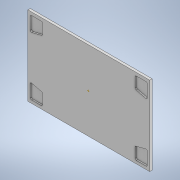
# Autodesk Inventor part: enclosuret
Saved by Autodesk Inventor 2021 (Build 250183000, 183)
## iProperties
Created: 2020-12-16
Part Number: enclosuret
Material: Generic
Document SubType Name: Modeling
Designer: oskar
Density: 1 g/cm^3
Appearance: Default
Author: oskar
Autodesk Inventor part; units mm, degrees
ref_plane "YZ Plane" through (0, 0, 0) normal (1, 0, 0) x (0, 1, 0)
ref_plane "XZ Plane" through (0, 0, 0) normal (0, 1, 0) x (-1, 0, 0)
ref_plane "XY Plane" through (0, 0, 0) normal (0, 0, 1) x (1, 0, 0)
ref_plane "Work Plane1" through (-0.485, 4.902, 12.06) normal (0, 0, 1) x (1, 0, 0)
sketch "Sketch1" plane through (-0.485, 4.902, 12.06) normal (0, 0, 1) x (1, 0, 0)
  line L0 (-52.815, 27.598) -> (47.185, 27.598)
  line L1 (47.185, 27.598) -> (47.185, -37.402)
  line L2 (47.185, -37.402) -> (-52.815, -37.402)
  line L3 (-52.815, -37.402) -> (-52.815, 27.598)
  line L4 (-52.815, 27.598) -> (47.185, -37.402) construction
  line L5 (47.185, 27.598) -> (-52.815, -37.402) construction
  line L6 (46.185, -13.982) -> (46.185, -20.322) projected
  line L7 (0.485, -4.902) -> (-19.0054, -4.902) construction
  point P0 (-2.815, -4.902)
  point P1 (-2.815, -4.902)
  dimension "d0" = 100
  dimension "d1" = 65
  dimension "d2" = 1
  constraints: 14 end point, 3 midpoint, 2 horizontal, 2 parallel, 1 perpendicular, 1 point on line
  measures "d0" distance of L0.start L0.end
  measures "d1" distance of L2.end L0.start
  measures "d2" distance between parallel lines of L6 L1
extrude "Extrusion1" add sketch "Sketch1" along normal blind 2
sketch "Sketch2" plane through (-0.485, 4.902, 14.06) normal (0, 0, 1) x (1, 0, 0)
  line L0 (36.185, 25.098) -> (44.185, 25.098)
  line L1 (45.185, 24.098) -> (45.185, 14.0681)
  line L2 (43.9425, 13.098) -> (35.9425, 15.098)
  line L3 (35.185, 16.0681) -> (35.185, 24.098)
  arc A0 (36.185, 25.098) -> (35.185, 24.098) centre (36.185, 24.098) ccw
  arc A1 (45.185, 24.098) -> (44.185, 25.098) centre (44.185, 24.098) ccw
  arc A2 (43.9425, 13.098) -> (45.185, 14.0681) centre (44.185, 14.0681) ccw
  arc A3 (35.185, 16.0681) -> (35.9425, 15.098) centre (36.185, 16.0681) ccw
  line L4 (-2.815, -4.902) -> (-2.815, 4.2729) construction
  line L5 (-2.815, -4.902) -> (-9.8185, -4.902) construction
  line L6 (-41.815, 25.098) -> (-49.815, 25.098)
  line L7 (-50.815, 24.098) -> (-50.815, 14.0681)
  line L8 (-49.5725, 13.098) -> (-41.5725, 15.098)
  line L9 (-40.815, 16.0681) -> (-40.815, 24.098)
  arc A4 (-40.815, 24.098) -> (-41.815, 25.098) centre (-41.815, 24.098) ccw
  arc A5 (-49.815, 25.098) -> (-50.815, 24.098) centre (-49.815, 24.098) ccw
  arc A6 (-50.815, 14.0681) -> (-49.5725, 13.098) centre (-49.815, 14.0681) ccw
  arc A7 (-41.5725, 15.098) -> (-40.815, 16.0681) centre (-41.815, 16.0681) ccw
  line L10 (36.185, -34.902) -> (44.185, -34.902)
  line L11 (45.185, -33.902) -> (45.185, -23.8721)
  line L12 (43.9425, -22.902) -> (35.9425, -24.902)
  line L13 (35.185, -25.8721) -> (35.185, -33.902)
  arc A8 (35.185, -33.902) -> (36.185, -34.902) centre (36.185, -33.902) ccw
  arc A9 (44.185, -34.902) -> (45.185, -33.902) centre (44.185, -33.902) ccw
  arc A10 (45.185, -23.8721) -> (43.9425, -22.902) centre (44.185, -23.8721) ccw
  arc A11 (35.9425, -24.902) -> (35.185, -25.8721) centre (36.185, -25.8721) ccw
  line L14 (-41.815, -34.902) -> (-49.815, -34.902)
  line L15 (-50.815, -33.902) -> (-50.815, -23.8721)
  line L16 (-49.5725, -22.902) -> (-41.5725, -24.902)
  line L17 (-40.815, -25.8721) -> (-40.815, -33.902)
  arc A12 (-41.815, -34.902) -> (-40.815, -33.902) centre (-41.815, -33.902) ccw
  arc A13 (-50.815, -33.902) -> (-49.815, -34.902) centre (-49.815, -33.902) ccw
  arc A14 (-49.5725, -22.902) -> (-50.815, -23.8721) centre (-49.815, -23.8721) ccw
  arc A15 (-40.815, -25.8721) -> (-41.5725, -24.902) centre (-41.815, -25.8721) ccw
  line L18 (47.185, -37.402) -> (47.185, 27.598) projected
  line L19 (-52.815, -37.402) -> (47.185, -37.402) projected
  point P0 (0.485, -4.902)
  dimension "d5" = 1
  dimension "d6" = 10
  dimension "d7" = 10
  dimension "d8" = 12
  dimension "d9" = 60
  dimension "d10" = 96
  dimension "d11" = 2
  dimension "d12" = 2.5
  constraints: 36 end point, 36 symmetric about line, 32 point on circle, 16 centre point, 8 tangent, 3 equal radius, 2 horizontal, 1 parallel, 1 perpendicular, 1 vertical, 12 other
  measures "d5" radius of A0
  measures "d6" distance between parallel lines of L3 L1
  measures "d7" distance from line of L2.end L0
  measures "d8" distance from line of L2.start L0
  measures "d9" distance between parallel lines of L0 L10
  measures "d10" distance between parallel lines of L7 L1
  measures "d11" distance between parallel lines of L18 L11
  measures "d12" distance between parallel lines of L19 L10
extrude "Extrusion2" cut sketch "Sketch2" against normal blind 1.2
body "Solid1"
